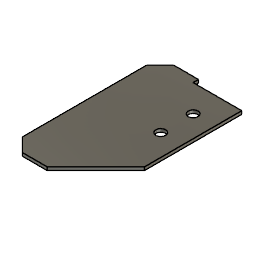
GPL H300 to H200G15 (Autodesk Fusion 360 design; units mm, degrees)
Autodesk Fusion 360 part; units mm, degrees
sketch "スケッチ1" plane through (0, 0, 0) normal (0, 0, 1) x (1, 0, 0)
  line L0 (-9.5, 140) -> (-80.5, 140)
  line L1 (-80.5, 140) -> (-80.5, -140)
  line L2 (-80.5, -140) -> (-9.5, -140)
  line L3 (80.5, -50) -> (80.5, 130)
  line L4 (74.75, 130) -> (-80.5, -140) construction
  line L5 (-80.5, 140) -> (47.6429, -82.8571) construction
  line L6 (-9.5, 140) -> (-9.5, 130)
  line L7 (-9.5, 130) -> (80.5, 130)
  line L8 (-80.5, -140) -> (-9.5, -140) construction
  line L9 (80.5, -50) -> (-9.5, -140)
  dimension "d2" = 280
  dimension "d5" = 71
  constraint horizontal L0
  constraint perpendicular L0 L1
  constraint parallel L0 L2
  constraint parallel L1 L3
  constraint coincident L4 origin
  constraint coincident L5 origin
  constraint vertical L6
  constraint horizontal L7
  constraint coincident L7 L4.start
  constraint perpendicular L1 L8
  constraint coincident L9 L5.end
  measures "d2" distance of L0.end L1.end
  measures "d5" distance of L1.end L2.end
extrude "押し出し1" add sketch "スケッチ1" along normal blind 6
chamfer "面取り1" distance 25 angle 45 2 edges at (-80.5, -140, 3) (-80.5, 140, 3)
sketch "スケッチ2" plane through (0, 0, 6) normal (0, 0, 1) x (-1, 0, 0)
  line L0 (55.5, -140) -> (80.5, -115)
  line L1 (80.5, -115) -> (80.5, 115)
  line L2 (80.5, 115) -> (55.5, 140)
  line L3 (55.5, 140) -> (9.5, 140)
  line L4 (9.5, 140) -> (-80.5, 50)
  line L5 (-80.5, 50) -> (-80.5, -130)
  line L6 (-80.5, -130) -> (9.5, -130)
  line L7 (9.5, -130) -> (9.5, -140)
  line L8 (9.5, -140) -> (55.5, -140)
  line L9 (-80.5, -130) -> (-40.5, -130) construction
  line L10 (-40.5, -130) -> (-40.5, -80) construction
  line L11 (-40.5, -80) -> (-80.5, -80) construction
  line L12 (-80.5, -80) -> (-80.5, -130) construction
  line L13 (-40.5, -80) -> (-40.5, -20) construction
  point P0 (-40.5, -80)
  point P1 (-40.5, -20)
  dimension "d10" = 40
  dimension "d11" = 50
  dimension "d12" = 60
  constraint horizontal L9
  constraint vertical L10
  constraint horizontal L11
  constraint vertical L12
  constraint coincident L5.end L6.start
  constraint perpendicular L11 L13
  constraint coincident P0 L10.end
  constraint coincident P1 L13.end
  measures "d10" distance of L5.end L9.end
  measures "d11" distance of L5.end L11.end
  measures "d12" distance of P0 P1
hole "穴1" at (40.5, 80, 6) at (40.5, 20, 6) direction (0, 0, -1) diameter 18 end through all
equation "d5 = 25 mm + 46 mm"
